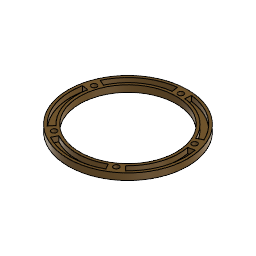
Ring (Autodesk Fusion 360 design; units mm, degrees)
part number: 2026-05-19-16-03-05-097
Autodesk Fusion 360 part; units mm, degrees
sketch "Sketch1" plane through (0, 0, 0) normal (0, 0, 1) x (1, 0, 0)
  circle A0 centre (0, 0) radius 54.5
  circle A1 centre (0, 0) radius 67.5
  line L0 (0, 0) -> (67.5, 0) construction
  line L1 (0, 0) -> (67.5, 0) construction
  line L2 (0, 56.25) -> (0, 63.25) construction
  circle A2 centre (0, 59.75) radius 3
  line L3 (-7.1543, 57.0532) -> (-8.2283, 63.973)
  line L4 (7.0818, 57.0622) -> (7.7138, 64.0371)
  line L5 (-56.4716, 10.8263) -> (-63.3846, 11.9432)
  circle A3 centre (-56.8256, 18.4638) radius 3
  line L6 (-52.081, 24.3683) -> (-58.5192, 27.1248)
  line L7 (-27.7471, -50.3622) -> (-30.9456, -56.5917)
  circle A4 centre (-35.1202, -48.3388) radius 3
  line L8 (-39.2696, -42.0018) -> (-43.8806, -47.273)
  line L9 (39.323, -41.9518) -> (44.2592, -46.9188)
  circle A5 centre (35.1202, -48.3388) radius 3
  line L10 (27.8111, -50.3269) -> (31.3995, -56.3411)
  line L11 (52.05, 24.4345) -> (58.2993, 27.5943)
  circle A6 centre (56.8256, 18.4638) radius 3
  line L12 (56.4578, 10.8981) -> (63.2866, 12.4523)
  arc A7 (52.05, 24.4345) -> (7.0818, 57.0622) centre (0, 0) ccw
  arc A8 (58.2993, 27.5943) -> (7.7138, 64.0371) centre (0, 0) ccw
  arc A9 (-7.1543, 57.0532) -> (-52.081, 24.3683) centre (0, 0) ccw
  arc A10 (-8.2283, 63.973) -> (-58.5192, 27.1248) centre (0, 0) ccw
  arc A11 (-56.4716, 10.8263) -> (-39.2696, -42.0018) centre (0, 0) ccw
  arc A12 (-63.3846, 11.9432) -> (-43.8806, -47.273) centre (0, 0) ccw
  arc A13 (-27.7471, -50.3622) -> (27.8111, -50.3269) centre (0, 0) ccw
  arc A14 (39.323, -41.9518) -> (56.4578, 10.8981) centre (0, 0) ccw
  arc A15 (-30.9456, -56.5917) -> (31.3995, -56.3411) centre (0, 0) ccw
  arc A16 (44.2592, -46.9188) -> (63.2866, 12.4523) centre (0, 0) ccw
  line L13 (0, 0) -> (0, 67.5) construction
  dimension "d1" = 109
  dimension "d2" = 135
  dimension "d3" = 115
  dimension "d4" = 129
  dimension "d7" = 6
  dimension "d8" = 7
  dimension "d10" = 360
  dimension "d11" = 59.75
  dimension "d12" = 14
  dimension "d14" = 7.2954
  dimension "d15" = 14.8681
  constraint coincident A0.centre A1.centre
  constraint concentric A1 A11
  constraint concentric A11 A12
  constraint horizontal L0
  constraint horizontal L1
  constraint vertical L2
  constraint midpoint L2 A2.centre
  constraint concentric A7 A9
  constraint concentric A8 A10
  constraint concentric A9 A11
  constraint concentric A10 A12
  constraint concentric A11 A13
  constraint concentric A12 A15
  constraint concentric A13 A14
  constraint concentric A15 A16
  constraint coincident L0.end L1.end
  constraint parallel L2 L13
  constraint coincident A2.centre L13
  constraint coincident A1 L13.end
  measures "d1" diameter of A0
  measures "d2" diameter of A1
  measures "d3" diameter of A9
  measures "d4" diameter of A10
  measures "d7" diameter of A2
  measures "d8" distance of L2.start L2.end
  measures "d11" vertical distance of A2.centre A0.centre
  measures "d12" angle of L3 L4
  measures "d14" distance of A2.centre L4
  measures "d15" horizontal distance of L4.end L3.start
extrude "Extrude1" add sketch "Sketch1" along normal blind 1.5 contours A2 | L3 L6 A9 A10 | L4 L11 A7 A8 | L5 L8 A11 A12 | A3 | L7 L10 A13 A15 | A4 | L9 L12 A14 A16 | A5 | A6 makes body 1 at (34.6202, -46.3461, 0) makes body 2 at (61.3877, 8.8614, 0) makes body 3 at (-54.8723, 28.9138, 0) makes body 4 at (-44.4551, -43.2519, 0) makes body 5 at (59.8219, 18.3142, 1) makes body 6 at (-53.8294, 18.3142, 1) makes body 7 at (27.3976, -55.6449, 0) makes body 8 at (10.5421, 61.1215, 0) makes body 9 at (-34.2393, -47.0468, 0) makes body 10 at (2.9963, 59.6005, 1)
extrude "Extrude2" add sketch "Sketch1" along normal blind 7.5 bodies 1 2 3 4 5 6 7 8 9 10
